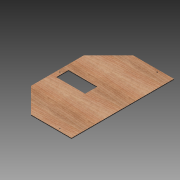
# Autodesk Inventor part: eLECTORNICS bOARD
Saved by Autodesk Inventor 2015 (Build 190159000, 159)
## iProperties
Created: 2015-02-07
Part Number: eLECTORNICS bOARD
Material: Generic
Document SubType Name: Modeling
Designer: pltwe4
Density: 1 g/cm^3
Appearance: Walnut
Author: pltwe4
Autodesk Inventor part; units mm, degrees
ref_plane "YZ Plane" through (0, 0, 0) normal (1, 0, 0) x (0, 1, 0)
ref_plane "XZ Plane" through (0, 0, 0) normal (0, 1, 0) x (-1, 0, 0)
ref_plane "XY Plane" through (0, 0, 0) normal (0, 0, 1) x (1, 0, 0)
sketch "Sketch7" plane through (0, 0, 0) normal (0, 1, 0) x (-1, 0, 0)
  line L0 (-204.851, 320.802) -> (-204.851, -320.802)
  line L1 (-204.851, -320.802) -> (49.149, -320.802)
  line L2 (204.851, -165.1) -> (204.851, 165.1)
  line L3 (49.149, 320.802) -> (-204.851, 320.802)
  line L4 (-286.7914, 0) -> (286.7914, 0) projected
  line L5 (0, -449.1228) -> (0, 449.1228) projected
  line L6 (172.847, -38.1) -> (-7.493, -38.1)
  line L7 (-7.493, -38.1) -> (-7.493, 38.1)
  line L8 (-7.493, 38.1) -> (172.847, 38.1)
  line L9 (172.847, 38.1) -> (172.847, -38.1)
  circle A0 centre (188.849, 0) radius 3.175
  circle A1 centre (-115.951, 304.8) radius 3.175
  circle A2 centre (-115.951, -304.8) radius 3.175
  line L10 (-27.051, -320.802) -> (-27.051, 320.802) construction
  line L11 (204.851, -70.0665) -> (-27.051, -70.0665) construction
  line L12 (204.851, 0) -> (143.8291, 0) construction
  line L13 (49.149, -320.802) -> (204.851, -165.1)
  line L14 (204.851, 165.1) -> (49.149, 320.802)
  point P0 (0, 0)
  dimension "d22" = 76.2
  dimension "d23" = 180.34
  dimension "d24" = 32.004
  dimension "d25" = 6.35
  dimension "d26" = 16.002
  dimension "d27" = 16.002
  dimension "d28" = 165.1
  dimension "d29" = 641.604
  dimension "d31" = 330.2
  dimension "d32" = 254
  dimension "d36" = 45
  dimension "d37" = 220.1959
  dimension "d38" = 231.902
  constraints: 26 end point, 5 parallel, 5 point on line, 4 perpendicular, 3 centre point, 2 horizontal, 1 collinear, 1 equal radius, 1 midpoint, 1 vertical, 4 other
  measures "d22" distance between parallel lines of L8 L6
  measures "d23" distance between parallel lines of L9 L7
  measures "d24" distance between parallel lines of L2 L9
  measures "d25" diameter of A2
  measures "d26" distance from line of L9 A0.centre
  measures "d27" distance from line of L1 A2.centre
  measures "d28" horizontal distance of L1.end A2.centre
  measures "d29" distance of L10.start L10.end
  measures "d31" distance of L2.start L2.end
  measures "d32" distance of L0.end L1.end
  measures "d36" angle of L2 L13
  measures "d37" distance of L1.end L2.start
  measures "d38" distance of L11.start L11.end
extrude "Extrusion5" add sketch "Sketch7" along normal blind 5.08 contours L3 L5 L8 L7 L4 L0 | L4 L7 L6 L5 L1 L0 | L3 L14 L2 L4 A0 L9 L8 L5 | L5 L6 L9 L4 A0 L2 L13 L1
equation "\"d28\" = 0.5 * SideLength"
equation "\"d31\" = SideLength"
equation "\"SideLength\" = 330.2"
body "Solid2"
